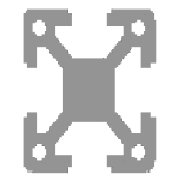
# Autodesk Inventor part: 420 mm
Saved by Autodesk Inventor 2016 (Build 200138000, 138)
## iProperties
IsCustomPart: 1
Created: 2023-12-31
Part Number: 420 mm
Material: Aluminum 6061
Description: ALU PROFILE 3030
Document SubType Name: Modeling
Standard: Aluminum Profile 30x30
Designer: Riskinova Oktavia
Standard Revision: Aluminum Profile 30x30
Manufacturer: Aluminum Profile 30x30
Standards Organization: Aluminum Profile 30x30
Language: en-US
Size Designation: (Unnamed 1)
Categories: <MemberInstance><Categories><Category DisplayName="Structural Shapes" InternalName="089c4875-fa83-4c05-b084-43b9cc11f5ed" Mnemonic="GRDR"><CategoryParameter DisplayName="Mass per Length Unit" InternalName="0bb95a10-148f-4027-a459-38d7b056702a" Mnemonic="shpmass"/><CategoryParameter DisplayName="Section Area" InternalName="1ff91680-64b0-4202-b9a3-7fd3f94bba3b" Mnemonic="secarea"/><CategoryParameter DisplayName="Radius of Gyration (x)" InternalName="25778675-03e9-40c1-b6a8-4a9ed693320d" Mnemonic="gyrradx"/><CategoryParameter DisplayName="Torsional Rigidity Modulus" InternalName="26c1ec35-5026-4c63-ad0a-751cf684a536" Mnemonic="torrigmod"/><CategoryParameter DisplayName="Distance of the Center of Gravity X-X" InternalName="26c9bdb8-9c79-4b4f-a92e-8e197583c9c4" Mnemonic="grcendistX"/><CategoryParameter DisplayName="Legacy Member ID" InternalName="340afe4f-75d7-48d3-ab7d-943f3c3da468" Mnemonic="LegacyMemberID"/><CategoryParameter DisplayName="Base Length" InternalName="42e34263-8f20-4d0e-ad48-bf1385b87c24" Mnemonic="shplen"/><CategoryParameter DisplayName="Moment of Inertia (y)" InternalName="4b9f58ea-bced-460e-81ea-3d29ca5a49e3" Mnemonic="inermomy"/><CategoryParameter DisplayName="Moment of Inertia (x)" InternalName="4cd780bc-73d7-43ac-917a-579e5cbd684d" Mnemonic="inermomx"/><CategoryParameter DisplayName="Custom Base Point" InternalName="4f1d1b73-316d-484b-a3df-9cbabb16eb77" Mnemonic="shpBasePoint"/><CategoryParameter DisplayName="Shape Height" InternalName="50274e7d-5ac0-4796-92cb-c59e54983c67" Mnemonic="shpheig"/><CategoryParameter DisplayName="Section Module (y)" InternalName="59eaa5e9-d227-48dc-b6c1-6920f96e0f95" Mnemonic="secmody"/><CategoryParameter DisplayName="Section Designation" InternalName="5a64d034-428d-49c8-ba32-7619764de20f" Mnemonic="shpdes"/><CategoryParameter DisplayName="Section Module (x)" InternalName="72cfad18-cf51-4ed4-aaa7-c6b224f8419f" Mnemonic="secmodx"/><CategoryParameter DisplayName="Torsional Section Modulus" InternalName="7c55a8dc-8844-49f9-a867-cc677b30ec9a" Mnemonic="torsecmod"/><CategoryParameter DisplayName="Shape Width" InternalName="7c717d54-a18f-4666-b4d4-573cce22c62c" Mnemonic="shpwdth"/><CategoryParameter DisplayName="Second Shape Thickness" InternalName="9251a8e1-85fd-4e47-af99-afdb762317d9" Mnemonic="shpthick2"/><CategoryParameter DisplayName="FG Authored" InternalName="9c666724-f362-4ea7-ac62-f6a007de5c69" Mnemonic="shpFGAuto"/><CategoryParameter DisplayName="Distance of the Center of Gravity Y-Y" InternalName="bcc4fb17-7af4-436a-8f8c-d0aa3b0248c5" Mnemonic="grcendistY"/><CategoryParameter DisplayName="Radius of Gyration (y)" InternalName="bfa18ebe-1636-4dbe-8d42-b263e0b73184" Mnemonic="gyrrady"/><CategoryParameter DisplayName="Shape Thickness" InternalName="d109cf76-8eb4-42fc-9800-4409734adc67" Mnemonic="shpthick"/><CategoryParameter DisplayName="Coefficient of Shear Displacement" InternalName="de4c90c6-aaa8-468f-a335-6737b311b5d3" Mnemonic="shdispc"/><Category DisplayName="Other" InternalName="f02205ff-2390-476f-921c-0b3185f88e84" Mnemonic="OTHSHP"><CategoryParameter DisplayName="Moment of Inertia (y)" InternalName="044c654e-f649-48ac-84cc-650a29ae31ca" Mnemonic="inermomy"/><CategoryParameter DisplayName="Shape Thickness" InternalName="12b1a788-9233-48fd-a933-2df8ff42b15f" Mnemonic="shpthick"/><CategoryParameter DisplayName="Mass per Length Unit" InternalName="2fd289d6-9394-4d2d-97e6-6659d7d4551d" Mnemonic="shpmass"/><CategoryParameter DisplayName="Radius of Gyration (y)" InternalName="743e1dfe-1bba-408b-b985-cf752b207386" Mnemonic="gyrrady"/><CategoryParameter DisplayName="Section Module (y)" InternalName="88b8bff9-a616-4028-93d5-ed4f79680d13" Mnemonic="secmody"/><CategoryParameter DisplayName="Section Area" InternalName="c46ecdf8-b6eb-4db9-8b25-30258930c1e3" Mnemonic="secarea"/><CategoryParameter DisplayName="Section Module (x)" InternalName="cac70804-9d39-43bb-be17-56ea1f39a6c2" Mnemonic="secmodx"/><CategoryParameter DisplayName="Moment of Inertia (x)" InternalName="ec6737bc-264f-43ed-b0bd-f6d410c2718d" Mnemonic="inermomx"/><CategoryParameter DisplayName="Radius of Gyration (x)" InternalName="ee72c61e-565e-4fd6-b448-66e1e1abcb7e" Mnemonic="gyrradx"/></Category></Category><Category DisplayName="DataType" InternalName="23b78d0f-2648-40c6-8793-ca6db495c9e8" Mnemonic="DATATYPE"><CategoryParameter DisplayName="DisplayName" InternalName="05415f3d-3907-474b-a020-eb9d644f4cf3" Mnemonic="DISPLAYNAME"/><CategoryParameter DisplayName="Standard" InternalName="0c0a119c-1e12-4c84-803f-101930972f5e" Mnemonic="STANDARD"/><CategoryParameter DisplayName="Description" InternalName="13903e3d-64b1-4950-80da-f627842ea37f" Mnemonic="DESCRIPTION"/><CategoryParameter DisplayName="Designation" InternalName="2675968c-4ce5-49e0-a4f5-552d29089031" Mnemonic="DESIGNATION"/><CategoryParameter DisplayName="Default Row" InternalName="2af9ec52-faaa-4026-b378-f9fa4afca842" Mnemonic="DEFAULTROW"/><CategoryParameter DisplayName="Folder Name" InternalName="3f06958e-8713-4116-9be7-ed6184ecc97b" Mnemonic="FOLDERNAME"/><CategoryParameter DisplayName="Revision Guid" InternalName="45a75005-10b1-4dfc-8d6d-dfe629f0b93c" Mnemonic="REVISIONGUID"/><CategoryParameter DisplayName="FileName" InternalName="8b46a4cc-9585-4fed-90c3-899f57e09a73" Mnemonic="FILENAME"/><CategoryParameter DisplayName="StdsOrg" InternalName="8f5914e1-4693-403f-8ab5-d37768198c9d" Mnemonic="STDSORG"/><CategoryParameter DisplayName="Family Version" InternalName="914462f6-6e19-4b14-ba84-155b9680b1d0" Mnemonic="FAMILYREVISION"/><CategoryParameter DisplayName="Standard Revision" InternalName="91d5a463-65c2-4fde-b823-3b7fea5e8e17" Mnemonic="STANDARDREVISION"/><CategoryParameter DisplayName="Member Revision" InternalName="a65d44b9-392f-4f4f-857b-e4b3d54996fe" Mnemonic="MEMBERREVISION"/><CategoryParameter DisplayName="ClipFormat" InternalName="bc51e27b-3422-4e78-93ef-cec197ddf230" Mnemonic="CLIPFORMAT"/><CategoryParameter DisplayName="Manufacturer" InternalName="cd6c7a72-a28a-4e50-99a9-2c7f4e13e5ad" Mnemonic="MANUFACTURER"/><CategoryParameter DisplayName="InternalName" InternalName="cf1d0246-76d9-4b4a-8305-fa0409afb5c1" Mnemonic="INTERNALNAME"/><CategoryParameter DisplayName="IsMetric" InternalName="e2385c5b-1ea4-4823-96a8-8de651266ec3" Mnemonic="ISMETRIC"/><Category DisplayName="Part" InternalName="c0e0b642-3bcb-4cc8-9e80-f96d35c4afa4" Mnemonic="PART"><CategoryParameter DisplayName="Part Number" InternalName="016b6077-bfbe-49bd-92c9-d8d59c39c941" Mnemonic="PARTNUMBER"/><CategoryParameter DisplayName="Stock Number" InternalName="4dba7c1c-e26c-444e-836c-b08b433409a8" Mnemonic="STOCKNUMBER"/><CategoryParameter DisplayName="Material Key" InternalName="5c9a8adb-dd2b-4535-b97f-0a94a95fe41f" Mnemonic="MATERIALKEY"/><CategoryParameter DisplayName="Material" InternalName="818a152a-d3c3-49ca-80ee-df7d91421b8e" Mnemonic="MATERIAL"/></Category></Category></Categories><FamilyTemplate Id="Aluminum Profile 30x30"><FamilyTemplateParameters><FamilyTemplateParameter ObjectType="kUserParameterObject" ValueType="xs:double" Id="1" ObjectReferenceKey="Length"/><FamilyTemplateParameter ObjectType="kUserParameterObject" ValueType="xs:double" Id="3" ObjectReferenceKey="X"/><FamilyTemplateParameter ObjectType="kUserParameterObject" ValueType="xs:double" Id="4" ObjectReferenceKey="Y"/><FamilyTemplateParameter ObjectType="kPartComponentDefinitionObject" ValueType="xs:string" Id="6" SubObjectId="Material"/><FamilyTemplateParameter ObjectType="kPropertyObject" ValueType="xs:string" Id="19" ObjectReferenceKey="{32853F0F-3444-11d1-9E93-0060B03C1CA6}" SubObjectId="5"/><FamilyTemplateParameter ObjectType="kPropertyObject" ValueType="xs:string" Id="20" ObjectReferenceKey="{32853F0F-3444-11d1-9E93-0060B03C1CA6}" SubObjectId="52"/></FamilyTemplateParameters></FamilyTemplate><CategoryParameterMap><ParamToTemplateMap><ParamToTemplate CategoryParameter="//CategoryParameter[@InternalName='cf1d0246-76d9-4b4a-8305-fa0409afb5c1']" ConstantValue="775c64f4-cae4-47e4-b8a8-46738fc38791"/><ParamToTemplate CategoryParameter="//CategoryParameter[@InternalName='45a75005-10b1-4dfc-8d6d-dfe629f0b93c']" ConstantValue="f9a7f22a-09ce-4afe-8c66-6e15ca7498bd"/><ParamToTemplate CategoryParameter="//CategoryParameter[@InternalName='3f06958e-8713-4116-9be7-ed6184ecc97b']" ConstantValue="Aluminum Profile 30x30"/><ParamToTemplate CategoryParameter="//CategoryParameter[@InternalName='8f5914e1-4693-403f-8ab5-d37768198c9d']" ConstantValue="Aluminum Profile 30x30"/><ParamToTemplate CategoryParameter="//CategoryParameter[@InternalName='0c0a119c-1e12-4c84-803f-101930972f5e']" ConstantValue="Aluminum Profile 30x30"/><ParamToTemplate CategoryParameter="//CategoryParameter[@InternalName='91d5a463-65c2-4fde-b823-3b7fea5e8e17']" ConstantValue="Aluminum Profile 30x30"/><ParamToTemplate CategoryParameter="//CategoryParameter[@InternalName='cd6c7a72-a28a-4e50-99a9-2c7f4e13e5ad']" ConstantValue="Aluminum Profile 30x30"/><ParamToTemplate CategoryParameter="//CategoryParameter[@InternalName='13903e3d-64b1-4950-80da-f627842ea37f']" ConstantValue="Aluminum Profile 30x30"/><ParamToTemplate CategoryParameter="//CategoryParameter[@InternalName='05415f3d-3907-474b-a020-eb9d644f4cf3']" ConstantValue="Aluminum Profile 30x30"/><ParamToTemplate CategoryParameter="//CategoryParameter[@InternalName='914462f6-6e19-4b14-ba84-155b9680b1d0']" ConstantValue="11"/><ParamToTemplate CategoryParameter="//CategoryParameter[@InternalName='bc51e27b-3422-4e78-93ef-cec197ddf230']" ConstantValue="CF_INVENTOR.STDPARTS"/><ParamToTemplate CategoryParameter="//CategoryParameter[@InternalName='e2385c5b-1ea4-4823-96a8-8de651266ec3']" ConstantValue="true"/><ParamToTemplate CategoryParameter="//CategoryParameter[@InternalName='2af9ec52-faaa-4026-b378-f9fa4afca842']" ConstantValue="1"/><ParamToTemplate CategoryParameter="//CategoryParameter[@InternalName='9c666724-f362-4ea7-ac62-f6a007de5c69']" ConstantValue="1"/><ParamToTemplate CategoryParameter="//CategoryParameter[@InternalName='8b46a4cc-9585-4fed-90c3-899f57e09a73']" ConstantValue="Aluminum Profile 30x30-01"/><ParamToTemplate CategoryParameter="//CategoryParameter[@InternalName='a65d44b9-392f-4f4f-857b-e4b3d54996fe']" ConstantValue="d43cdd5c-9d0c-4519-a97f-b06fbdebb047"/><ParamToTemplate CategoryParameter="//CategoryParameter[@InternalName='a65d44b9-392f-4f4f-857b-e4b3d54996fe']" ConstantValue="d43cdd5c-9d0c-4519-a97f-b06fbdebb047"/><ParamToTemplate CategoryParameter="//CategoryParameter[@InternalName='2675968c-4ce5-49e0-a4f5-552d29089031']" TemplateParameter="20"/><ParamToTemplate CategoryParameter="//CategoryParameter[@InternalName='42e34263-8f20-4d0e-ad48-bf1385b87c24']" TemplateParameter="1"/><ParamToTemplate CategoryParameter="//CategoryParameter[@InternalName='818a152a-d3c3-49ca-80ee-df7d91421b8e']" TemplateParameter="6"/><ParamToTemplate CategoryParameter="//CategoryParameter[@InternalName='016b6077-bfbe-49bd-92c9-d8d59c39c941']" TemplateParameter="19"/></ParamToTemplateMap></CategoryParameterMap></MemberInstance>
Density: 2.7 g/cm^3
Appearance: Aluminum - Flat
_CCFamilyMember: 1
_CCFamilyDisplayName: Aluminum Profile 30x30 - Aluminum Profile 30x30
_FrameMemberDoc: Frame Member File
_Version: 15.0.0
_GetPNFromCC: 1
X: 30.000 mm
Y: 30.000 mm
Length: 450.000 mm
G_L: 420.000 mm
G_W: 30.000 mm
G_H: 30.000 mm
+2F9365F7-9515-466F-ADC2-AE1075E03174+CUTDETAIL1: Cut
+02611102-B929-442C-8C02-B3FFFD9BB060+CUTDETAIL2: Cut
Author: Riskinova Oktavia
Autodesk Inventor part; units mm, degrees
ref_plane "YZ Plane" through (0, 0, 0) normal (1, 0, 0) x (0, 1, 0)
ref_plane "XZ Plane" through (0, 0, 0) normal (0, 1, 0) x (-1, 0, 0)
ref_plane "Work Plane3" through (0, 0, 250) normal (0, 0, 1) x (1, 0, 0)
sketch "Sketch2" plane through (0, 0, 250) normal (0, 0, 1) x (1, 0, 0)
  circle A0 centre (0, 0) radius 3.4
  dimension "d51" = 6.8
  constraints: 1 centre point, 1 coincident
  measures "d51" diameter of A0
extrude "Extrusion2" [suppressed]
ref_plane "Start Plane" through (0, 0, 15) normal (0, 0, 1) x (1, 0, 0)
ref_plane "End Plane" through (0, 0, 435) normal (0, 0, 1) x (1, 0, 0)
sketch "Sketch" plane through (0, 0, 0) normal (0, 0, 1) x (1, 0, 0)
  line L0 (-13, 15) -> (13, 15)
  line L1 (15, 13) -> (15, -13)
  line L2 (-15, 15) -> (15, -15) construction
  line L3 (15, 15) -> (-15, -15) construction
  line L4 (-5.2, 15) -> (-5.2, 14.2)
  line L5 (-5.2, 14.2) -> (-4.1, 14.2)
  line L6 (-4.1, 14.2) -> (-4.1, 12.2)
  line L7 (-4.1, 12.2) -> (-8.25, 12.2)
  line L8 (-8.25, 12.2) -> (-8.25, 10.2)
  line L9 (-8.25, 10.2) -> (-3.85, 5.8)
  line L10 (-3.85, 5.8) -> (3.85, 5.8)
  line L11 (8.25, 12.2) -> (4.1, 12.2)
  line L12 (4.1, 12.2) -> (4.1, 14.2)
  line L13 (4.1, 14.2) -> (5.2, 14.2)
  line L14 (5.2, 14.2) -> (5.2, 15)
  line L15 (8.25, 12.2) -> (8.25, 10.2)
  line L16 (8.25, 10.2) -> (3.85, 5.8)
  line L17 (-5.8, 0) -> (5.8, 0)
  line L18 (-5.2, -15) -> (-5.2, -14.2)
  line L19 (-5.2, -14.2) -> (-4.1, -14.2)
  line L20 (-4.1, -14.2) -> (-4.1, -12.2)
  line L21 (-4.1, -12.2) -> (-8.25, -12.2)
  line L22 (-8.25, -12.2) -> (-8.25, -10.2)
  line L23 (-8.25, -10.2) -> (-3.85, -5.8)
  line L24 (-3.85, -5.8) -> (3.85, -5.8)
  line L25 (8.25, -12.2) -> (4.1, -12.2)
  line L26 (4.1, -12.2) -> (4.1, -14.2)
  line L27 (4.1, -14.2) -> (5.2, -14.2)
  line L28 (5.2, -14.2) -> (5.2, -15)
  line L29 (8.25, -12.2) -> (8.25, -10.2)
  line L30 (8.25, -10.2) -> (3.85, -5.8)
  line L31 (0, 5.8) -> (0, -5.8)
  line L32 (15, 5.2) -> (14.2, 5.2)
  line L33 (14.2, 5.2) -> (14.2, 4.1)
  line L34 (14.2, 4.1) -> (12.2, 4.1)
  line L35 (12.2, 4.1) -> (12.2, 8.25)
  line L36 (15, -5.2) -> (14.2, -5.2)
  line L37 (14.2, -5.2) -> (14.2, -4.1)
  line L38 (14.2, -4.1) -> (12.2, -4.1)
  line L39 (12.2, -4.1) -> (12.2, -8.25)
  line L40 (12.2, -8.25) -> (10.2, -8.25)
  line L41 (10.2, -8.25) -> (5.8, -3.85)
  line L42 (5.8, -3.85) -> (5.8, 3.85)
  line L43 (5.8, 3.85) -> (10.2, 8.25)
  line L44 (10.2, 8.25) -> (12.2, 8.25)
  line L45 (-15, 5.2) -> (-14.2, 5.2)
  line L46 (-14.2, 5.2) -> (-14.2, 4.1)
  line L47 (-14.2, 4.1) -> (-12.2, 4.1)
  line L48 (-12.2, 4.1) -> (-12.2, 8.25)
  line L49 (-15, -5.2) -> (-14.2, -5.2)
  line L50 (-14.2, -5.2) -> (-14.2, -4.1)
  line L51 (-14.2, -4.1) -> (-12.2, -4.1)
  line L52 (-12.2, -4.1) -> (-12.2, -8.25)
  line L53 (-12.2, -8.25) -> (-10.2, -8.25)
  line L54 (-10.2, -8.25) -> (-5.8, -3.85)
  line L55 (-5.8, -3.85) -> (-5.8, 3.85)
  line L56 (-5.8, 3.85) -> (-10.2, 8.25)
  line L57 (-10.2, 8.25) -> (-12.2, 8.25)
  circle A0 centre (11.5, 11.5) radius 1.65
  circle A1 centre (11.5, -11.5) radius 1.65
  circle A2 centre (-11.5, 11.5) radius 1.65
  circle A3 centre (-11.5, -11.5) radius 1.65
  line L58 (-15, -13) -> (-15, -5.2)
  line L59 (-15, 5.2) -> (-15, 13)
  line L60 (13, -15) -> (5.2, -15)
  line L61 (-5.2, -15) -> (-13, -15)
  arc A4 (-13, 15) -> (-15, 13) centre (-13, 13) ccw
  arc A5 (15, 13) -> (13, 15) centre (13, 13) ccw
  arc A6 (13, -15) -> (15, -13) centre (13, -13) ccw
  arc A7 (-15, -13) -> (-13, -15) centre (-13, -13) ccw
  point P0 (0, 0)
  point P1 (0, 0)
  dimension "d2" = 8.2
  dimension "d3" = 4.1
  dimension "d4" = 10.4
  dimension "d5" = 5.2
  dimension "d8" = 9.2
  dimension "d11" = 16.5
  dimension "d12" = 8.25
  dimension "d14" = 0.8
  dimension "d15" = 2
  dimension "d16" = 2
  dimension "d34" = 0.8
  dimension "d35" = 10.4
  dimension "d36" = 5.2
  dimension "d37" = 8.2
  dimension "d38" = 4.1
  dimension "d39" = 2
  dimension "d40" = 16.5
  dimension "d41" = 8.25
  dimension "d42" = 2
  dimension "d43" = 9.2
  dimension "d44" = 23
  dimension "d45" = 11.5
  dimension "d46" = 23
  dimension "d47" = 11.5
  dimension "d48" = 3.3
  dimension "d55" = 2
  constraints: 124 end point, 28 symmetric about line, 20 point on line, 13 perpendicular, 11 parallel, 8 centre point, 8 point on circle, 8 tangent, 7 midpoint, 6 equal radius, 4 vertical alignment, 3 horizontal, 3 horizontal alignment, 2 collinear, 2 vertical
  measures "d2" distance between parallel lines of L12 L6
  measures "d3" distance from line of L31.start L6
  measures "d4" distance from line of L13.end L4
  measures "d5" distance from line of point (0, 0) L14
  measures "d8" distance between parallel lines of L10 L0
  measures "d11" distance between parallel lines of L8 L15
  measures "d12" distance from line of point (0, 0) L15
  measures "d14" distance of L13.end L14.end
  measures "d15" distance of L11.end L12.end
  measures "d16" distance of L11.start L15.end
  measures "d34" distance of L36.start L36.end
  measures "d35" distance between parallel lines of L36 L32
  measures "d36" distance from line of point (0, 0) L36
  measures "d37" distance between parallel lines of L34 L38
  measures "d38" distance from line of point (0, 0) L38
  measures "d39" distance of L37.end L38.end
  measures "d40" distance of L35.end L39.end
  measures "d41" vertical distance of point (0, 0) L39.end
  measures "d42" distance of L39.end L40.end
  measures "d43" distance between parallel lines of L42 L1
  measures "d44" distance of A1.centre A0.centre
  measures "d45" horizontal distance of point (0, 0) A1.centre
  measures "d46" distance of A3.centre A1.centre
  measures "d47" horizontal distance of point (0, 0) A1.centre
  measures "d48" diameter of A1
  measures "d55" radius of A4
extrude "Body" add sketch "Sketch" along normal up to surface (420 mm away) from surface at 15 contours L0 L4 L5 L6 L7 L8 L9 L10 L31 L17 L55 L56 L57 L48 L47 L46 L45 L59 A4 | L0 A5 L1 L32 L33 L34 L35 L44 L43 L42 L17 L31 L10 L16 L15 L11 L12 L13 L14 | L1 A6 L60 L28 L27 L26 L25 L29 L30 L24 L31 L17 L42 L41 L40 L39 L38 L37 L36 | L31 L24 L23 L22 L21 L20 L19 L18 L61 A7 L58 L49 L50 L51 L52 L53 L54 L55 L17
sketch "Sketch3" plane through (0, 0, 0) normal (0, 0, 1) x (1, 0, 0)
  line L0 (0, 0) -> (10, 0)
ref_plane "Work Plane4" through (0, 0, 0) normal (0, -1, 0) x (1, 0, 0)
sketch "Sketch4" plane through (0, 0, 0) normal (0, -1, 0) x (1, 0, 0)
  line L0 (-2, 15) -> (12, 15)
  line L1 (-2, 435) -> (12, 435)
  dimension "d61" = 420
  measures "d61" distance between parallel lines of L0 L1
ref_plane "Work Plane5" through (-185, 5.2, 435) normal (0, 0, 1) x (1, 0, 0)
split "Split1" plane through (-185, 5.2, 435) removes the side toward (0, 0, 1)
ref_plane "Work Plane6" through (265, 5.2, 15) normal (0, 0, -1) x (-1, 0, 0)
split "Split2" plane through (265, 5.2, 15) removes the side toward (0, 0, -1)
equation "\"d3\" = 0.5 * d2"
equation "\"d5\" = 0.5 * d4"
equation "\"d12\" = 0.5 * d11"
equation "\"d36\" = 0.5 * d35"
equation "\"d38\" = 0.5 * d37"
equation "\"d41\" = 0.5 * d40"
equation "\"d45\" = 0.5 * d44"
equation "\"d47\" = 0.5 * d46"
equation "\"G_OFFSET_START\" = -15"
equation "\"G_OFFSET_END\" = -15"
equation "\"d56\" = -G_OFFSET_START"
equation "\"G_L\" = d61"
body "Solid1"
